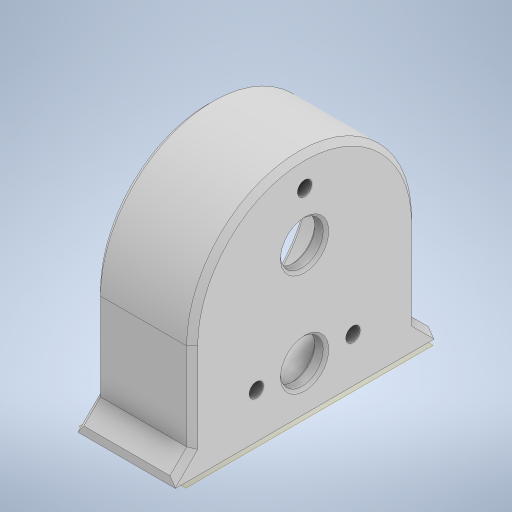
# Autodesk Inventor part: pump_socket
Saved by Autodesk Inventor 2024 (Build 280153000, 153)
## iProperties
Created: 2023-05-19
Part Number: pump_socket
Material: Generic
Document SubType Name: Modeling
Designer: jeff7
Density: 1 g/cm^3
Appearance: Default
Author: jeff7
Autodesk Inventor part; units mm, degrees
ref_plane "YZ Plane" through (0, 0, 0) normal (1, 0, 0) x (0, 1, 0)
ref_plane "XY Plane" through (0, 0, 0) normal (0, 0, 1) x (1, 0, 0)
sketch "Sketch1" plane through (0, 0, 0) normal (1, 0, 0) x (0, 1, 0)
  circle A0 centre (0, 0) radius 20.25
  circle A1 centre (0, 0) radius 17.25 construction
  circle A2 centre (6.1, 0) radius 3.85
  circle A3 centre (-12.35, 0) radius 3.85
  circle A4 centre (14.95, 0) radius 1.3
  circle A5 centre (-12.158, 8.7) radius 1.3
  circle A6 centre (-12.158, -8.7) radius 1.3
  dimension "d0" = 40.5
  dimension "d1" = 34.5
  dimension "d2" = 7.7
  dimension "d3" = 7.7
  dimension "d4" = 6.1
  dimension "d5" = 12.35
  dimension "d6" = 2.6
  dimension "d7" = 2.6
  dimension "d8" = 2.6
  dimension "d9" = 14.95
  dimension "d10" = 17.4
  dimension "d12" = 8.7
  dimension "d13" = 12.158
  constraints: 7 centre point, 3 horizontal alignment, 2 coincident, 1 vertical alignment
  measures "d0" diameter of A0
  measures "d1" diameter of A1
  measures "d2" diameter of A3
  measures "d3" diameter of A2
  measures "d4" distance of point (0, 0) A2.centre
  measures "d5" distance of point (0, 0) A3.centre
  measures "d6" diameter of A4
  measures "d7" diameter of A5
  measures "d8" diameter of A6
  measures "d9" distance of point (0, 0) A4.centre
  measures "d10" distance of A6.centre A5.centre
  measures "d12" vertical distance of point (0, 0) A5.centre
  measures "d13" horizontal distance of point (0, 0) A5.centre
extrude "Extrusion1" add sketch "Sketch1" against normal blind 2.5
sketch "Sketch2" plane through (-2.5, 0, 0) normal (-1, 0, 0) x (0, 0, 1)
  circle A0 centre (0, 0) radius 17.25
  circle A1 centre (0, 0) radius 20.25 projected
  dimension "d16" = 34.5
  constraints: 1 centre point, 1 coincident
  measures "d16" diameter of A0
extrude "Extrusion2" add sketch "Sketch2" along normal blind 15
ref_plane "Work Plane1" through (0, -20.25, 0) normal (0, 1, 0) x (-1, 0, 0)
sketch "Sketch3" plane through (0, -20.25, 0) normal (0, 1, 0) x (-1, 0, 0)
  line L0 (0, 20.25) -> (17.5, 20.25) projected
  line L1 (0, 20.25) -> (0, -20.25) projected
  line L2 (17.5, -20.25) -> (17.5, 20.25) projected
  line L3 (0, -20.25) -> (17.5, -20.25) projected
  point P0 (0, 0)
extrude "Extrusion3" add sketch "Sketch3" along normal up to surface round surface about axis through (0, 0, 0) along (-1, 0, 0) radius 20.25 far side no
sketch "Sketch4" plane through (0, -20.25, 0) normal (0, 1, 0) x (-1, 0, 0)
  line L0 (0, 20.25) -> (17.5, 20.25) projected
  line L1 (17.5, 20.25) -> (0, 20.25)
  line L2 (0, 20.25) -> (0, 23.25)
  line L3 (0, 23.25) -> (17.5, 23.25)
  line L4 (17.5, 23.25) -> (17.5, 20.25)
  line L5 (0, 20.25) -> (0, -20.25) projected
  line L6 (0, -20.25) -> (17.5, -20.25)
  line L7 (17.5, -20.25) -> (17.5, -23.25)
  line L8 (17.5, -23.25) -> (0, -23.25)
  line L9 (0, -23.25) -> (0, -20.25)
  point P0 (0, 0)
  dimension "d21" = 3
  dimension "d22" = 3
  constraints: 16 end point, 4 parallel, 2 horizontal, 2 perpendicular
  measures "d21" distance between parallel lines of L0 L3
  measures "d22" distance between parallel lines of L8 L6
extrude "Extrusion4" add sketch "Sketch4" along normal blind 3
chamfer "Chamfer1" distance 1.5 angle 45 4 edges at (-8.75, -17.25, 20.25) (-8.75, -17.25, 23.25) (-8.75, -17.25, -20.25) (-8.75, -17.25, -23.25)
chamfer "Chamfer2" distance 1 angle 45 20 edges at (0, 14.3189, -14.3189) (0, 14.3189, 14.3189) (0, -7.8751, 20.25) (0, -7.8751, -20.25) (-17.5, 20.25, 0) (-17.5, -7.8751, -20.25) (-17.5, -7.8751, 20.25) (0, -16.5001, 21) (0, -18, 22.5) (0, -17.25, 21.75) (0, -16.5001, -21) (0, -17.25, -21.75) (0, -18, -22.5) (-17.5, -16.5001, 21) (-17.5, -18, 22.5) (-17.5, -17.25, 21.75) (-17.5, -16.5001, -21) (-17.5, -18, -22.5) (-17.5, -17.25, -21.75) (-17.5, 0, -17.25)
chamfer "Chamfer3" distance 0.5 angle 45 4 edges at (-2.5, 2.25, 0) (-2.5, -16.2, 0) (0, 2.25, 0) (0, -16.2, 0)
equation "\"d1\" = dia_pump"
equation "\"d2\" = dia_hose"
equation "\"d3\" = dia_hose"
equation "\"d6\" = dia_screw"
equation "\"d7\" = dia_screw"
equation "\"d8\" = dia_screw"
equation "\"wall_thick\" = 3"
equation "\"dia_pump\" = 34.5"
equation "\"dia_hose\" = 7.7"
equation "\"dia_screw\" = 2.6"
body "Solid1"
